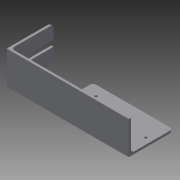
# Autodesk Inventor part: LaserMount
Saved by Autodesk Inventor 2015 (Build 190159000, 159)
## iProperties
Created: 2015-09-05
Part Number: LaserMount
Material: Generic
Document SubType Name: Modeling
Designer: Kurtis
Density: 1 g/cm^3
Appearance: Default
Author: Kurtis
Autodesk Inventor part; units mm, degrees
ref_plane "YZ Plane" through (0, 0, 0) normal (1, 0, 0) x (0, 1, 0)
ref_plane "XZ Plane" through (0, 0, 0) normal (0, 1, 0) x (-1, 0, 0)
ref_plane "XY Plane" through (0, 0, 0) normal (0, 0, 1) x (1, 0, 0)
sketch "Sketch1" plane through (0, 0, 0) normal (0, 0, 1) x (1, 0, 0)
  line L0 (0, 0) -> (104, 0)
  line L1 (104, 0) -> (104, 54.5)
  line L2 (104, 54.5) -> (0, 54.5)
  line L3 (0, 54.5) -> (0, 10)
  circle A0 centre (96, 27.25) radius 1.625
  circle A1 centre (17, 41.25) radius 1.625
  circle A2 centre (17, 13.25) radius 1.625
  line L4 (0, 0) -> (-10, 0)
  line L5 (-10, 0) -> (-10, 10)
  line L6 (-10, 10) -> (0, 10)
  dimension "d0" = 104
  dimension "d1" = 54.5
  dimension "d9" = 28
  dimension "d10" = 13.25
  dimension "d11" = 17
  dimension "d12" = 3.25
  dimension "d13" = 3.25
  dimension "d14" = 17
  dimension "d15" = 8
  dimension "d16" = 3.25
  dimension "d17" = 27.25
  dimension "d34" = 10
  dimension "d35" = 10
  constraints: 14 end point, 4 perpendicular, 3 centre point, 2 horizontal, 1 parallel, 1 vertical
  measures "d0" distance of L0.start L0.end
  measures "d1" distance of L0.end L1.end
  measures "d9" distance of A2.centre A1.centre
  measures "d10" distance from line of A2.centre L0
  measures "d11" distance from line of A2.centre L3
  measures "d12" diameter of A2
  measures "d13" diameter of A1
  measures "d14" distance from line of L3 A1.centre
  measures "d15" distance from line of L1 A0.centre
  measures "d16" diameter of A0
  measures "d17" distance from line of L0 A0.centre
  measures "d34" distance of L0.start L4.end
  measures "d35" distance of L4.end L5.end
extrude "Main Mount" add sketch "Sketch1" along normal blind 3
sketch "Sketch2" plane through (0, 0, 0) normal (0, -1, 0) x (1, 0, 0)
  line L0 (104, 0) -> (0, 0)
  line L1 (0, 0) -> (104, 0) projected
  line L2 (0, 0) -> (-55, 0)
  line L3 (-55, 0) -> (-55, 43)
  line L4 (-55, 43) -> (104, 43)
  line L5 (104, 43) -> (104, 0)
  line L6 (104, 0) -> (0, 0)
  dimension "d20" = 55
  dimension "d21" = 43
  constraints: 12 end point, 3 perpendicular, 2 collinear, 1 point on line
  measures "d20" distance of L0.end L2.end
  measures "d21" distance of L2.end L3.end
extrude "Base" add sketch "Sketch2" along normal blind 3
sketch "Sketch3" plane through (0, 0, 0) normal (0, 1, 0) x (1, 0, 0)
  line L0 (-55, 0) -> (-52, 0)
  line L1 (-55, 0) -> (104, 0) projected
  line L2 (-52, -43) -> (-55, -43)
  line L3 (-55, -43) -> (-55, 0)
  line L4 (-55, -43) -> (-55, 0) projected
  line L5 (-52, -17.5) -> (-55, -17.5)
  line L6 (-55, -43) -> (-55, 0) projected
  line L7 (-52, -25.5) -> (-55, -25.5)
  line L8 (-52, 0) -> (-52, -17.5)
  line L9 (-52, -25.5) -> (-52, -43)
  dimension "d24" = 3
  dimension "d31" = 8
  constraints: 14 end point, 5 perpendicular, 3 point on line, 2 equal length, 1 collinear
  measures "d24" distance of L0.start L0.end
  measures "d31" distance between parallel lines of L7 L5
extrude "Laser Mount" add sketch "Sketch3" along normal blind 55
hole "Cable Management" at (-5, 5, 3) direction (0, 0, -1) diameter 6.5 depth 8 tip angle 118
hole "Cable Routing" at (-52, 5, 5) direction (-1, 0, 0) diameter 4 depth 8 tip angle 118
fillet "Strength" radius 4 10 edges at (-52, 0, 8.75) (-52, 0, 34.25) (-53.5, 55, 43) (-53.5, 55, 0) (47, 0, 3) (-10, 0, 1.5) (-10, 10, 1.5) (0, 10, 1.5) (0, 54.5, 1.5) (104, 54.5, 1.5)
body "Solid1"
